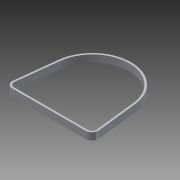
# Autodesk Inventor part: Clippard Zip Tie 2
Saved by Autodesk Inventor 2014 SP1 (Build 180222100, 222)
## iProperties
Created: 2013-12-13
Part Number: Clippard Zip Tie 2
Material: ABS Plastic
Document SubType Name: Modeling
Designer: Moses
Mass: 1.38224 g
Surface Area: 25.6692 cm^2
Volume: 1.304 cm^3
Density: 1.06 g/cm^3
Appearance: Smooth - White
Author: Moses
Autodesk Inventor part; units mm, degrees
ref_plane "YZ Plane" through (0, 0, 0) normal (1, 0, 0) x (0, 1, 0)
ref_plane "XZ Plane" through (0, 0, 0) normal (0, 1, 0) x (-1, 0, 0)
ref_plane "XY Plane" through (0, 0, 0) normal (0, 0, 1) x (1, 0, 0)
sketch "Sketch1" plane through (0, 0, 0) normal (0, 1, 0) x (-1, 0, 0)
  line L0 (0, 0) -> (52.3748, 0) construction
  arc A0 (52.2043, -29.1712) -> (0.1705, -29.1712) centre (26.1874, -26.1874) ccw construction
  line L1 (0, 0) -> (-6.35, 0) construction
  line L2 (52.3748, 0) -> (58.7248, 0) construction
  line L3 (0, 0) -> (0, -26.1874) construction
  line L4 (52.3748, 0) -> (52.3748, -26.1874) construction
  line L5 (-3.175, 0) -> (0.1705, -29.1712)
  line L6 (55.5498, 0) -> (52.2043, -29.1712)
  arc A1 (0.1705, -29.1712) -> (52.2043, -29.1712) centre (26.1874, -26.1874) ccw
  line L7 (-0.0207, 3.5368) -> (52.3955, 3.5368)
  arc A2 (-0.0207, 3.5368) -> (-3.175, 0) centre (-0.0207, 0.3618) ccw
  arc A3 (55.5498, 0) -> (52.3955, 3.5368) centre (52.3955, 0.3618) ccw
  arc A4 (56.8115, -0.1447) -> (52.3955, 4.8068) centre (52.3955, 0.3618) ccw
  line L8 (52.3955, 4.8068) -> (-0.0207, 4.8068)
  arc A5 (-0.0207, 4.8068) -> (-4.4367, -0.1447) centre (-0.0207, 0.3618) ccw
  line L9 (-4.4367, -0.1447) -> (-1.0912, -29.3159)
  arc A6 (-1.0912, -29.3159) -> (53.466, -29.3159) centre (26.1874, -26.1874) ccw
  line L10 (56.8115, -0.1447) -> (53.466, -29.3159)
  dimension "d0" = 52.3748
  dimension "d1" = 52.3748
  dimension "d2" = 6.35
  dimension "d3" = 6.35
  dimension "d4" = 3.175
  dimension "d5" = 1.27
  dimension "d6" = 1.27
  dimension "d7" = 1.27
  dimension "d8" = 1.27
  constraints: 22 end point, 16 point on circle, 9 tangent, 7 centre point, 4 horizontal, 2 midpoint, 2 parallel, 1 vertical, 2 other
  measures "d0" distance of L0.start L0.end
  measures "d1" diameter of A0
  measures "d2" distance of L0.start L1.end
  measures "d3" distance of L0.end L2.end
  measures "d4" radius of A2
  measures "d5" distance between parallel lines of L7 L8
  measures "d6" radial gap between concentric circles of A1 A6
  measures "d7" distance between parallel lines of L5 L9
  measures "d8" distance between parallel lines of L10 L6
extrude "Extrusion1" add sketch "Sketch1" along normal blind 5.08
body "Solid1"
